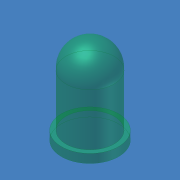
# Autodesk Inventor part: LED - Green
Saved by Autodesk Inventor 2014 SP1 (Build 180222100, 222)
## iProperties
Shininess: 64.0
Length Units: 11272
Angle Units: 11279
Time Units: 11290
Mass Units: 11286
Length Display Precision: 3
Angle Display Precision: 2
Compacted: True
Part Number: LED - Green
Document SubType Name: Modeling
Created: 2005-12-27
Designer: Owner
Material: ABS Plastic
Density: 1 g/cm^3
Appearance: Green (Clear)
Density: 0.0
Volumn: 0.0
Area: 0.0
PropertySet Name: Model Information
Control State: 0
Master: False
Checked Out: False
Author: Owner
Autodesk Inventor part; units mm, degrees
ref_plane "YZ Plane" through (0, 0, 0) normal (1, 0, 0) x (0, 1, 0)
ref_plane "XZ Plane" through (0, 0, 0) normal (0, 1, 0) x (-1, 0, 0)
ref_plane "XY Plane" through (0, 0, 0) normal (0, 0, 1) x (1, 0, 0)
sketch "Sketch1" plane through (0, 0, 0) normal (0, 0, 1) x (1, 0, 0)
  line L0 (0, 0) -> (0, 9)
  arc A0 (0, 9) -> (-2.4915, 6.277) centre (-0.0014, 6.5) ccw
  line L1 (-2.4915, 6.277) -> (-2.4915, 0.9)
  line L2 (-2.4915, 0.9) -> (-2.95, 0.9)
  line L3 (-2.95, 0.9) -> (-2.95, 0)
  line L4 (-2.95, 0) -> (0, 0)
  dimension "d0" = 5
  dimension "d1" = 9
  dimension "d2" = 0.9
  dimension "d3" = 2.95
  constraints: 10 end point, 3 parallel, 2 point on circle, 1 centre point, 1 perpendicular, 1 vertical, 1 other
  measures "d0" diameter of A0
  measures "d1" distance of L0.start L0.end
  measures "d2" distance of L2.end L3.end
  measures "d3" distance of L3.end L0.start
revolve "Revolution1" add sketch "Sketch1" angle 360 about axis through (0, 0, 0) along (0, 1, 0)
body "Solid1"
